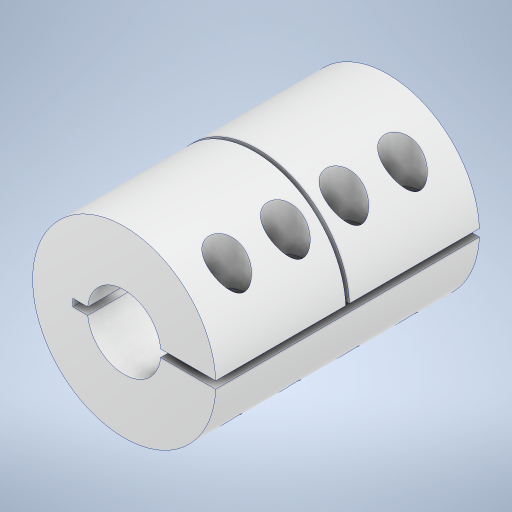
# Autodesk Inventor part: coupling
Saved by Autodesk Inventor 2023 (Build 270158000, 158)
## iProperties
Created: 2023-05-28
Part Number: coupling
Material: Aluminum 6061
Document SubType Name: Modeling
Designer: 310611102
Density: 2.7 g/cm^3
Appearance: Aluminum - Flat
Mass: 36.9035 g
Surface Area: 63.8687 cm^2
Volume: 13.668 cm^3
Author: 310611102
Autodesk Inventor part; units mm, degrees
ref_plane "YZ Plane" through (0, 0, 0) normal (1, 0, 0) x (0, 1, 0)
ref_plane "XY Plane" through (0, 0, 0) normal (0, 0, 1) x (1, 0, 0)
sketch "Sketch1" plane through (0, 0, 0) normal (0, 0, 1) x (1, 0, 0)
  circle A0 centre (0, 0) radius 12.5
  circle A1 centre (0, 0) radius 5
  dimension "d0" = 25
  dimension "d1" = 10
  constraints: 2 centre point, 2 coincident
  measures "d0" diameter of A0
  measures "d1" diameter of A1
extrude "Extrusion1" add sketch "Sketch1" along normal blind 36
sketch "Sketch3" plane through (0, 0, 36) normal (0, 0, 1) x (1, 0, 0)
  line L0 (-7, 0.5) -> (12.5, 0.5)
  line L1 (12.5, 0.5) -> (12.5, -0.5)
  line L2 (12.5, -0.5) -> (-7, -0.5)
  line L3 (-7, -0.5) -> (-7, 0.5)
  line L4 (-7, 0.5) -> (12.5, -0.5) construction
  line L5 (12.5, 0.5) -> (-7, -0.5) construction
  circle A0 centre (0, 0) radius 12.5 projected
  point P0 (-7, 0)
  point P1 (2.75, 0)
  point P2 (-7, 0)
  point P3 (12.5, 0)
  point P4 (12.49, -0.5)
  point P5 (12.49, 0.5)
  dimension "d7" = 1
  dimension "d10" = 7
  constraints: 12 end point, 4 midpoint, 2 parallel, 1 coincident, 1 horizontal, 1 horizontal alignment, 1 perpendicular, 2 other
  measures "d7" distance of L0.end L1.end
  measures "d10" distance from line of L3 point (0, 0)
extrude "Extrusion3" cut sketch "Sketch3" against normal through all contours L0 A0 L2 L3 picked at (-0.5, 0)
sketch "Sketch4" plane through (0, 0, 0) normal (1, 0, 0) x (0, 1, 0)
  line L0 (30, 18.25) -> (0, 18.25)
  line L1 (0, 18.25) -> (0, 17.75)
  line L2 (0, 17.75) -> (30, 17.75)
  line L3 (30, 17.75) -> (30, 18.25)
  line L4 (30, 18.25) -> (0, 17.75) construction
  line L5 (0, 18.25) -> (30, 17.75) construction
  line L6 (12.5, 0) -> (-12.5, 0) projected
  point P0 (0, 0)
  point P1 (15, 18)
  point P2 (0.5, 0)
  point P3 (-0.5, 0)
  point P4 (15, 18.25)
  dimension "d11" = 0.5
  dimension "d12" = 0
  dimension "d13" = 30
  dimension "d18" = 18
  constraints: 12 end point, 3 midpoint, 2 parallel, 1 horizontal, 1 perpendicular
  measures "d11" distance of L2.end L0.start
  measures "d12" distance from line of point (0, 0) L1
  measures "d13" distance of L1.end L2.end
  measures "d18" distance from line of L6 point (15, 18)
extrude "Extrusion4" cut sketch "Sketch4" along normal through all both and the other way through all
ref_plane "Work Plane1" through (0, 12.5, 0) normal (0, 1, 0) x (-1, 0, 0)
sketch "Sketch5" plane through (0, 12.5, 0) normal (0, 1, 0) x (-1, 0, 0)
  circle A0 centre (-7.995, 22) radius 2.4
  line L0 (14.0583, 18) -> (-17.4822, 18)
  line L1 (12.5, 0) -> (-12.49, 0) projected
  circle A1 centre (-7.995, 30) radius 2.4
  line L2 (12.5, 36) -> (-12.49, 36) projected
  circle A2 centre (-7.995, 14) radius 2.4
  circle A3 centre (-7.995, 6) radius 2.4
  point P0 (0, 0)
  point P1 (0.005, 36)
  dimension "d17" = 18
  dimension "d19" = 4.8
  dimension "d20" = 4.8
  dimension "d21" = 8
  dimension "d22" = 6
  dimension "d23" = 8
  constraints: 4 centre point, 2 end point, 2 symmetric about line, 1 horizontal, 1 midpoint, 1 vertical alignment, 2 other
  measures "d17" distance between parallel lines of L1 L0
  measures "d19" diameter of A0
  measures "d20" diameter of A1
  measures "d21" distance of A0.centre A1.centre
  measures "d22" distance from line of L2 A1.centre
  measures "d23" horizontal distance of point (0.005, 36) A0.centre
extrude "Extrusion5" cut sketch "Sketch5" against normal blind 8
sketch "Sketch6" plane through (0, 12.5, 0) normal (0, 1, 0) x (-1, 0, 0)
  circle A0 centre (-7.995, 30) radius 2.4 projected
  circle A1 centre (-7.995, 30) radius 1.5
  circle A2 centre (-7.995, 22) radius 2.4 projected
  circle A3 centre (-7.995, 22) radius 1.5
  circle A4 centre (-7.995, 14) radius 2.4 projected
  circle A5 centre (-7.995, 14) radius 1.5
  circle A6 centre (-7.995, 6) radius 2.4 projected
  circle A7 centre (-7.995, 6) radius 1.5
  point P0 (0, 0)
  dimension "d26" = 3
  constraints: 4 centre point, 4 coincident, 3 equal radius
  measures "d26" diameter of A1
extrude "Extrusion6" cut sketch "Sketch6" against normal through all contours A1 | A3 | A5 | A7
sketch "Sketch2" plane through (0, 0, 0) normal (0, 1, 0) x (-1, 0, 0)
  circle A0 centre (0, 5.5789) radius 1.6
  line L0 (16.8162, 18) -> (-14.2715, 18)
  line L1 (12.5, 36) -> (-12.5, 36) projected
  line L2 (12.5, 0) -> (-12.5, 0) projected
  line L3 (12.5, 36) -> (12.5, 18)
  line L4 (12.5, 18) -> (12.5, 0)
  circle A1 centre (0, 30.4211) radius 1.6
  point P0 (0, 0)
  dimension "d4" = 3.2
  constraints: 6 end point, 2 centre point, 2 collinear, 1 horizontal, 1 point on line, 1 symmetric about line, 1 other
  measures "d4" diameter of A0
equation "\"d20\" = d19"
body "Solid1"
